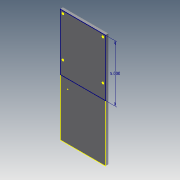
# Autodesk Inventor part: kinect rotate side
Saved by Autodesk Inventor 2011 (Build 150239000, 239)
## iProperties
Created: 2012-01-14
Part Number: kinect rotate side
Document SubType Name: Modeling
Designer: Matthew
Density: 1 g/cm^3
Author: Matthew
Autodesk Inventor part; units mm, degrees
ref_plane "YZ Plane" through (0, 0, 0) normal (1, 0, 0) x (0, 1, 0)
ref_plane "XZ Plane" through (0, 0, 0) normal (0, 1, 0) x (-1, 0, 0)
ref_plane "XY Plane" through (0, 0, 0) normal (0, 0, 1) x (1, 0, 0)
sketch "Sketch1" plane through (0, 0, 0) normal (0, 0, 1) x (1, 0, 0)
  line L0 (-17.3633, -106.383) -> (84.2367, -106.383)
  line L1 (84.2367, -106.383) -> (84.2367, 147.617)
  line L2 (84.2367, 147.617) -> (-17.3633, 147.617)
  line L3 (-17.3633, 147.617) -> (-17.3633, -106.383)
  line L4 (-17.3633, 147.617) -> (-11.3943, 147.617)
  line L5 (-11.3943, 147.617) -> (-11.3943, 141.648)
  line L6 (-11.3943, 141.648) -> (-17.3633, 141.648)
  line L7 (-17.3633, 141.648) -> (-17.3633, 147.617)
  line L8 (84.2367, 147.617) -> (78.2677, 147.617)
  line L9 (78.2677, 147.617) -> (78.2677, 141.648)
  line L10 (78.2677, 141.648) -> (84.2367, 141.648)
  line L11 (84.2367, 141.648) -> (84.2367, 147.617)
  line L12 (-11.3943, 141.648) -> (78.2677, 141.648)
  line L13 (78.2677, 141.648) -> (78.2677, 51.986)
  line L14 (78.2677, 51.986) -> (-11.3943, 51.986)
  line L15 (-11.3943, 51.986) -> (-11.3943, 141.648)
  circle A0 centre (-11.3943, 141.648) radius 1.9812
  circle A1 centre (78.2677, 141.648) radius 1.9812
  circle A2 centre (78.2677, 51.986) radius 1.9812
  circle A3 centre (-11.3943, 51.986) radius 1.9812
  point P0 (0, 0)
  dimension "d0" = 101.6
  dimension "d1" = 254
  dimension "d2" = 5.969
  dimension "d3" = 5.969
  dimension "d4" = 5.969
  dimension "d5" = 89.662
  dimension "d6" = 3.9624
  constraints: 32 end point, 8 parallel, 4 centre point, 4 coincident, 4 horizontal, 4 perpendicular
  measures "d0" distance of L2.end L1.end
  measures "d1" distance of L1.end L0.end
  measures "d2" distance of L5.end L6.end
  measures "d3" distance of L4.end L5.end
  measures "d4" distance of L10.end L9.end
  measures "d5" distance of L12.end L13.end
  measures "d6" diameter of A0
extrude "Extrusion1" add sketch "Sketch1" along normal blind 6.35 contours L3 L6 A0 L15 A3 L14 A2 L13 A1 L10 L1 L0 | L3 L2 L5 A0 L6 | L10 A1 L9 L2 L1 | A0 L5 L6 | L10 L9 A1 | L2 L9 A1 L12 A0 L5 | L12 A0 L15 | A0 L12 A1 L13 A2 L14 A3 L15 | L13 A1 L12 | A3 L14 L15 | L13 L14 A2 picked at (-10.4662, 52.9141) picked at (77.0289, 52.4195)
sketch "Sketch2" plane through (0, 0, 6.35) normal (0, 0, 1) x (1, 0, 0)
  line L0 (78.2677, 141.648) -> (78.2677, 143.6292) projected
  line L1 (80.2489, 141.648) -> (78.2677, 141.648) projected
  arc A0 (78.2677, 139.6668) -> (80.2489, 141.648) centre (78.2677, 141.648) ccw projected
  line L2 (78.2677, 141.648) -> (78.2677, 139.6668) projected
  line L3 (76.2865, 141.648) -> (78.2677, 141.648) projected
  arc A1 (78.2677, 143.6292) -> (76.2865, 141.648) centre (78.2677, 141.648) ccw projected
  line L4 (-11.3943, 143.6292) -> (-11.3943, 141.648) projected
  arc A2 (-9.4131, 141.648) -> (-11.3943, 143.6292) centre (-11.3943, 141.648) ccw projected
  line L5 (-11.3943, 141.648) -> (-9.4131, 141.648) projected
  line L6 (-11.3943, 139.6668) -> (-11.3943, 141.648) projected
  arc A3 (-13.3755, 141.648) -> (-11.3943, 139.6668) centre (-11.3943, 141.648) ccw projected
  line L7 (-11.3943, 141.648) -> (-13.3755, 141.648) projected
  arc A4 (-11.3943, 53.9672) -> (-9.4131, 51.986) centre (-11.3943, 51.986) ccw projected
  line L8 (-11.3943, 51.986) -> (-11.3943, 53.9672) projected
  line L9 (-9.4131, 51.986) -> (-11.3943, 51.986) projected
  line L10 (78.2677, 53.9672) -> (78.2677, 51.986) projected
  arc A5 (76.2865, 51.986) -> (78.2677, 53.9672) centre (78.2677, 51.986) ccw projected
  line L11 (78.2677, 51.986) -> (76.2865, 51.986) projected
  circle A6 centre (-11.3943, 141.648) radius 1.9812
  circle A7 centre (78.2677, 141.648) radius 1.9812
  circle A8 centre (78.2677, 51.986) radius 1.9812
  circle A9 centre (-11.3943, 51.986) radius 1.9812
  point P0 (0, 0)
  constraints: 4 coincident, 3 horizontal alignment, 1 vertical alignment, 8 other
extrude "Extrusion2" cut sketch "Sketch2" against normal blind 25.4 contours L0 A7 L1 | L2 A7 L3 | L4 L7 A6 | L5 A6 L6 | A9 L9 L8 | L10 L11 A8
sketch "Sketch3" plane through (0, 0, 6.35) normal (0, 0, 1) x (1, 0, 0)
  line L0 (-17.3633, 147.617) -> (84.2367, 147.617) projected
  line L1 (-17.3633, -106.383) -> (-17.3633, 147.617) projected
  line L2 (84.2367, -106.383) -> (-17.3633, -106.383) projected
  line L3 (84.2367, 147.617) -> (84.2367, -106.383) projected
  line L4 (-17.3633, 147.617) -> (84.2367, 147.617)
  line L5 (84.2367, 147.617) -> (84.2367, 20.617)
  line L6 (84.2367, 20.617) -> (-17.3633, 20.617)
  line L7 (-17.3633, 20.617) -> (-17.3633, 147.617)
  point P0 (0, 0)
  dimension "d11" = 127
  constraints: 8 end point, 2 parallel, 1 horizontal, 1 midpoint, 1 perpendicular
  measures "d11" distance of L4.end L5.end
extrude "Extrusion3" cut sketch "Sketch3" against normal blind 25.4 contours L6 L3 L2 L1
sketch "Sketch4" plane through (0, 0, 0) normal (0, 0, -1) x (-1, 0, 0)
  circle A0 centre (11.3943, 51.986) radius 1.9812 projected
  circle A1 centre (-78.2677, 51.986) radius 1.9812 projected
  line L0 (-84.2367, 20.617) -> (-84.2367, 147.617) projected
  circle A2 centre (11.3943, 141.648) radius 1.9812 projected
  circle A3 centre (-78.2677, 141.648) radius 1.9812 projected
  line L1 (-78.2677, 141.648) -> (11.3943, 51.986)
  line L2 (-78.2677, 51.986) -> (11.3943, 141.648)
  circle A4 centre (-33.4367, 96.817) radius 11.5
  line L3 (-33.4367, 96.817) -> (-43.9367, 96.817)
  line L4 (-43.9367, 96.817) -> (-22.9367, 96.817)
  line L5 (-22.9367, 96.817) -> (-22.9367, 61.817)
  line L6 (-22.9367, 61.817) -> (-43.9367, 61.817)
  line L7 (-43.9367, 61.817) -> (-43.9367, 96.817)
  point P0 (0, 0)
  dimension "d14" = 23
  dimension "d15" = 10.5
  dimension "d16" = 21
  dimension "d17" = 35
  constraints: 14 end point, 3 perpendicular, 2 parallel, 1 centre point, 1 horizontal, 1 midpoint
  measures "d14" diameter of A4
  measures "d15" distance of L3.start L3.end
  measures "d16" distance of L5.end L6.end
  measures "d17" distance of L4.end L5.end
extrude "Extrusion4" cut sketch "Sketch4" against normal blind 25.4 contours L5 L6 L7 L2 A4 L1 | L1 A4 L5 | A4 L2 L1 | L1 L4 L5 A4 | L5 L4 L2 A4 | L3 L7 A4 L1 | L1 A4 L2 | L2 A4 L7 L3 | L2 L7 A4
sketch "Sketch5" plane through (0, 0, 0) normal (0, 0, -1) x (-1, 0, 0)
  arc A0 (-22.9367, 92.1266) -> (-43.9367, 92.1266) centre (-33.4367, 96.817) ccw projected
  line L0 (-22.9367, 92.1266) -> (-22.9367, 61.817) projected
  line L1 (-84.2367, 20.617) -> (-84.2367, 147.617) projected
  line L2 (-33.4367, 96.817) -> (-46.9367, 96.817)
  line L3 (-46.9367, 96.817) -> (-46.9367, 90.317)
  line L4 (-46.9367, 90.317) -> (-19.9367, 90.317)
  line L5 (-46.9367, 90.317) -> (-19.9367, 90.317)
  line L6 (-19.9367, 90.317) -> (-19.9367, 74.317)
  line L7 (-19.9367, 74.317) -> (-46.9367, 74.317)
  line L8 (-46.9367, 74.317) -> (-46.9367, 90.317)
  circle A1 centre (-46.9367, 90.317) radius 1
  circle A2 centre (-19.9367, 90.317) radius 1
  circle A3 centre (-19.9367, 74.317) radius 1
  circle A4 centre (-46.9367, 74.317) radius 1
  point P0 (0, 0)
  dimension "d20" = 13.5
  dimension "d21" = 6.5
  dimension "d22" = 27
  dimension "d23" = 16
  dimension "d24" = 2
  constraints: 14 end point, 4 centre point, 4 coincident, 4 perpendicular, 2 parallel, 1 horizontal
  measures "d20" distance of L2.start L2.end
  measures "d21" distance of L2.end L3.end
  measures "d22" distance of L3.end L4.end
  measures "d23" distance of L5.end L6.end
  measures "d24" diameter of A1
extrude "Extrusion5" cut sketch "Sketch5" against normal blind 25.4 contours A1 L8 L4 | L4 L3 A1 | A2 L6 L4 | L4 L6 A2 | L3 L8 A1 | A3 L6 L7 | L7 L6 A3 | A4 L8 L7 | L7 L8 A4
body "Solid1"
